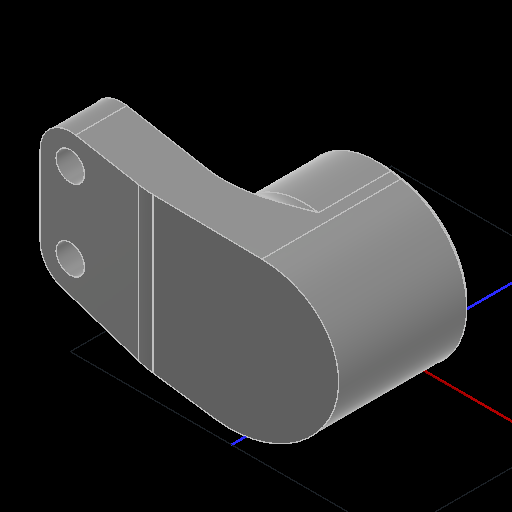
# Autodesk Inventor part: thing
Saved by Autodesk Inventor 2025.2 (Build 292293000, 293)
## iProperties
Created: 2025-11-17
Part Number: thing
Material: white pla
Document SubType Name: Modeling
Designer: cloudy
Density: 1 g/cm^3
Appearance: Smooth - Dark Gray
Author: cloudy
Autodesk Inventor part; units mm, degrees
ref_plane "YZ Plane" through (0, 0, 0) normal (1, 0, 0) x (0, 1, 0)
ref_plane "XZ Plane" through (0, 0, 0) normal (0, 1, 0) x (-1, 0, 0)
sketch "Sketch1" plane through (0, 0, 0) normal (0, 0, 1) x (1, 0, 0)
  arc A0 (-3.9687, -12.064) -> (2.2782, 12.494) centre (0, 0) ccw
  circle A1 centre (-25.4, 0) radius 2.2479
  circle A2 centre (-25.4, 12.7) radius 2.2479
  line L0 (-25.4, 0) -> (-25.4, 12.7) construction
  line L1 (0, 0) -> (-25.4, 0) construction
  arc A3 (-24.5457, 17.3852) -> (-30.1625, 12.7) centre (-25.4, 12.7) ccw
  arc A4 (-30.1625, 0) -> (-26.8883, -4.524) centre (-25.4, 0) ccw
  line L2 (-26.8883, -4.524) -> (-3.9687, -12.064)
  line L3 (2.2782, 12.494) -> (-24.5457, 17.3852)
  line L4 (-30.1625, 12.7) -> (-30.1625, 0)
  circle A5 centre (0, 0) radius 9.525
  dimension "d0" = 25.4
  dimension "d1" = 12.7
  dimension "d2" = 4.4958
  dimension "d3" = 25.4
  dimension "d8" = 9.525
  dimension "d9" = 9.525
  dimension "d10" = 19.05
  constraints: 10 end point, 6 centre point, 6 point on circle, 5 tangent, 4 coincident, 2 vertical, 1 equal radius, 1 horizontal
  measures "d0" diameter of A0
  measures "d1" distance of L0.start L0.end
  measures "d2" diameter of A2
  measures "d3" distance of L1.start L0.start
  measures "d8" diameter of A3
  measures "d9" diameter of A4
  measures "d10" diameter of A5
extrude "Extrusion1" add sketch "Sketch1" along normal blind 25.4
sketch "Sketch2" plane through (0, 0, 0) normal (0, 1, 0) x (-1, 0, 0)
  line L0 (-25.3065, 18.9574) -> (19.1186, 26.3269)
  line L1 (19.1186, 26.3269) -> (-25.6271, 26.3269)
  line L2 (-25.6271, 26.3269) -> (-25.3065, 18.9574)
  point P0 (0, 0)
  constraints: 6 end point
extrude "Extrusion2" cut sketch "Sketch2" along normal through all both and the other way through all
fillet "Fillet1" radius 12.7 1 edges at (-13.531, 3.2293, 25.4)
ref_plane "Work Plane1" through (0, 0, 19.05) normal (0, 0, -1) x (-1, 0, 0)
sketch "Sketch4" plane through (-30.1625, 0, 0) normal (-1, 0, 0) x (0, 0, 1)
  line L0 (17.3005, 18.8893) -> (-1.1849, 18.8893)
  line L1 (-1.1849, 18.8893) -> (-1.1849, -14.6789)
  line L2 (-1.1849, -14.6789) -> (17.3005, -14.6789)
  line L3 (17.3005, -14.6789) -> (17.3005, 18.8893)
  point P0 (0, 0)
  constraints: 8 end point, 2 parallel, 1 horizontal, 1 perpendicular
extrude "Extrusion4" cut sketch "Sketch4" against normal blind 15.875
fillet "Fillet2" radius 12.7 1 edges at (-14.2875, 15.5147, 8.6503)
fillet "Fillet3" radius 10.16 1 edges at (-14.2875, -8.6693, 8.6503)
fillet "Fillet4" radius 5.08 3 edges at (-12.358, -7.2729, 17.3005) (-9.7225, 10.042, 17.3005) (-14.2875, -0.5133, 17.3005)
sketch "Sketch6" plane through (0, 0, 19.05) normal (0, 0, -1) x (-1, 0, 0)
  circle A0 centre (0, 0) radius 9.525 projected
  arc A1 (7.3025, -10.9672) -> (14.2875, -1.3161) centre (4.1275, -1.3161) ccw projected
  line L0 (14.2875, -1.3161) -> (14.2875, 0.2895) projected
  arc A2 (14.2875, 0.2895) -> (-0.6907, 12.7835) centre (1.5875, 0.2895) ccw projected
  line L1 (-2.2782, 12.494) -> (-0.6907, 12.7835) projected
  arc A3 (-2.2782, 12.494) -> (3.9687, -12.064) centre (0, 0) ccw projected
  line L2 (7.3025, -10.9672) -> (3.9687, -12.064) projected
extrude "Extrusion6" add sketch "Sketch6" against normal up to surface contours A0 surface through (25.3065, 0, 18.9574) normal (-0.1636509, 0, -0.9865183)
chamfer "Chamfer1" distance 0.7937 angle 45 1 edges at (-9.525, 0, 19.05)
chamfer "Chamfer2" distance 0.7937 angle 45 6 edges at (-9.7225, 10.042, 0) (-14.2875, -0.5133, 0) (-12.358, -7.2729, 0) (-5.6356, -11.5156, 0) (12.308, -3.1309, 0) (1.4845, 12.6387, 0)
body "Solid1"
